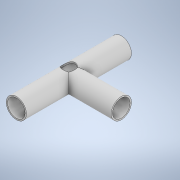
# Autodesk Inventor part: bar elbow
Saved by Autodesk Inventor 2021 (Build 250183000, 183)
## iProperties
Created: 2020-07-11
Part Number: bar elbow
Material: Generic
Document SubType Name: Modeling
Designer: Shannon
Density: 1 g/cm^3
Appearance: Default
Author: Shannon
Autodesk Inventor part; units mm, degrees
ref_plane "XY Plane" through (0, 0, 0) normal (0, 0, 1) x (1, 0, 0)
sketch "Sketch1" plane through (0, 0, 0) normal (0, 0, 1) x (1, 0, 0)
  circle A0 centre (0, 0) radius 7.366
  dimension "d0" = 14.732
  constraints: 1 centre point, 1 coincident
  measures "d0" diameter of A0
extrude "Extrusion1" add sketch "Sketch1" along normal blind 76.2
sketch "Sketch2" plane through (0, 0, 76.2) normal (0, 0, 1) x (1, 0, 0)
  circle A0 centre (0, 0) radius 7.366 projected
  circle A1 centre (0, 0) radius 6.35
  dimension "d3" = 12.7
  constraints: 1 centre point, 1 coincident
  measures "d3" diameter of A1
extrude "Extrusion2" cut sketch "Sketch2" against normal blind 76.2 contours A1
ref_plane "Work Plane1" through (38.1, 0, 0) normal (1, 0, 0) x (0, 1, 0)
sketch "Sketch3" plane through (38.1, 0, 0) normal (1, 0, 0) x (0, 1, 0)
  circle A0 centre (0, 38.1) radius 7.366
  line L0 (7.366, 76.2) -> (-7.366, 76.2) projected
  point P0 (0, 0)
  dimension "d7" = 14.732
  dimension "d8" = 38.1
  constraints: 1 centre point
  measures "d7" diameter of A0
  measures "d8" distance from line of L0 A0.centre
extrude "Extrusion3" add sketch "Sketch3" against normal up to surface round surface about axis through (0, 0, 0) along (0, 0, 1) radius 7.366 far side no
sketch "Sketch4" plane through (38.1, 0, 38.1) normal (1, 0, 0) x (0, 0, -1)
  circle A0 centre (0, 0) radius 6.35
  point P0 (38.1, 0)
  dimension "d11" = 12.7
  constraints: 1 centre point
  measures "d11" diameter of A0
extrude "Extrusion4" cut sketch "Sketch4" against normal up to surface round surface about axis through (0, 0, 0) along (0, 0, 1) radius 7.366 far side no
ref_plane "Work Plane2" through (0, 7.366, 0) normal (0, 1, 0) x (-1, 0, 0)
sketch "Sketch5" plane through (0, 7.366, 0) normal (0, 1, 0) x (-1, 0, 0)
  circle A0 centre (0, 38.1) radius 4.4608
  point P0 (0, 0)
  dimension "d14" = 38.1
  constraints: 1 centre point
  measures "d14" distance of A0.centre point (0, 0)
extrude "Extrusion5" cut sketch "Sketch5" against normal through all
body "Solid1"
